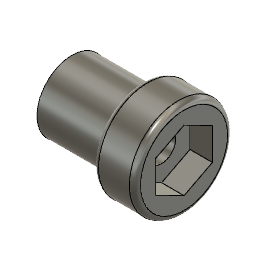
BearingPlug (Autodesk Fusion 360 design; units mm, degrees)
Autodesk Fusion 360 part; units mm, degrees
sketch "Sketch1" plane through (0, 0, 0) normal (1, 0, 0) x (0, 0, -1)
  circle A0 centre (0, 0) radius 2.5
  dimension "d1" = 5
  constraint coincident A0.centre origin
  measures "d1" diameter of A0
extrude "Extrude1" add sketch "Sketch1" along normal blind 5
sketch "Sketch2" plane through (5, 0, 0) normal (1, 0, 0) x (0, 0, -1)
  circle A0 centre (0, 0) radius 2.5
  circle A1 centre (0, 0) radius 3.5
  dimension "d4" = 7
  constraint coincident A0.centre A1.centre
  measures "d4" diameter of A1
extrude "Extrude2" add sketch "Sketch2" along normal blind 3 contours A0 | A1
sketch "Sketch3" plane through (0, 0, 0) normal (1, 0, 0) x (0, 0, -1)
  circle A0 centre (0, 0) radius 1
  dimension "d7" = 2
  constraint coincident A0.centre origin
  measures "d7" diameter of A0
extrude "Extrude3" cut sketch "Sketch3" along normal up to surface (8 mm away)
sketch "Sketch4" plane through (8, 0, 0) normal (1, 0, 0) x (0, 0, -1)
  circle A0 centre (0, 0) radius 1
  circle A1 centre (0, 0) radius 3.5
  line L0 (2.02, -2.1816) -> (-2.02, -2.1816) construction
  line L1 (-2.02, -2.1816) -> (-2.02, 2.1816) construction
  line L2 (-2.02, 2.1816) -> (2.02, 2.1816) construction
  line L3 (2.02, 2.1816) -> (2.02, -2.1816) construction
  line L4 (2.02, -2.1816) -> (-2.02, 2.1816) construction
  line L5 (-2.02, -2.1816) -> (2.02, 2.1816) construction
  line L6 (-2.02, 0) -> (2.02, 0) construction
  line L7 (0, -2.1816) -> (0, 2.1816) construction
  line L8 (-2.02, 1.137) -> (-2.02, -1.137)
  line L9 (2.02, 1.137) -> (2.02, -1.137)
  line L10 (-2.02, 1.137) -> (0, 2.1816)
  line L11 (0, 2.1816) -> (2.02, 1.137)
  line L12 (2.02, -1.137) -> (0, -2.1816)
  line L13 (0, -2.1816) -> (-2.02, -1.137)
  dimension "d10" = 4.04
  dimension "d11" = 4.3632
  constraint horizontal L0
  constraint perpendicular L0 L1
  constraint parallel L0 L2
  constraint parallel L1 L3
  constraint coincident L4 A0.centre
  constraint coincident L5 A0.centre
  constraint coincident A0.centre A1.centre
  constraint midpoint L1 L6.start
  constraint midpoint L3 L6.end
  constraint midpoint L0 L7.start
  constraint midpoint L2 L7.end
  constraint perpendicular L6 L8
  constraint perpendicular L2 L9
  constraint equal L8 L9
  constraint midpoint L6.start L8
  constraint midpoint L6.end L9
  constraint equal L8 L10
  measures "d10" distance of L1.end L2.end
  measures "d11" distance of L0.end L1.end
extrude "Extrude4" cut sketch "Sketch4" against normal blind 1.6 contours L8 L9 L10 L11 L12 L13
fillet "Fillet1" radius 0.3 1 edges at (5, -0.904, 2.3308)
fillet "Fillet2" radius 0.4 2 edges at (5, -1.2657, 3.2631) (8, -1.2657, 3.2631)
sketch "Sketch5" plane through (0, 0, 0) normal (1, 0, 0) x (0, 0, -1)
  line L0 (-3.5, 0) -> (3.5, 0)
  line L1 (3.5, 0) -> (3.5, -3.5)
  line L2 (3.5, -3.5) -> (-3.5, -3.5)
  line L3 (-3.5, -3.5) -> (-3.5, 0)
  dimension "d18" = 7
  dimension "d19" = 3.5
  constraint horizontal L0
  constraint vertical L1
  constraint horizontal L2
  constraint vertical L3
  constraint midpoint origin L0
  measures "d18" distance of L0.start L0.end
  measures "d19" distance of L0.end L1.end
extrude "Extrude5" [rolled back] side1offset 0 taper angle 0
equation "d10 = ( 4 * 1.01 ) * 1 mm"
equation "d11 = ( 4.32 * 1.01 ) * 1 mm"
